Autodesk Fusion 360 part; units mm, degrees
note: some values were not read from the file. Set by a fixed rule: which sketch regions a step uses.
(part 2 of 59)
  spline S4 degree 5 poles (13.0527, -15.6181) (13.0525, -15.6154) (13.0521, -15.61) (13.0515, -15.6019) (13.0506, -15.5911) (13.0495, -15.5777) (13.0484, -15.5644) (13.0473, -15.551) (13.0462, -15.5377) (13.0451, -15.5244) (13.0439, -15.5112) (13.0427, -15.4979) (13.0415, -15.4848) (13.0404, -15.4716) (13.0391, -15.4585) (13.0379, -15.4454) (13.0367, -15.4323) (13.0354, -15.4193) (13.0342, -15.4063) (13.0329, -15.3934) (13.0316, -15.3805) (13.0303, -15.3676) (13.029, -15.3547) (13.0276, -15.3419) (13.0263, -15.3291) (13.0249, -15.3164) (13.0236, -15.3037) (13.0222, -15.291) (13.0208, -15.2784) (13.0194, -15.2658) (13.018, -15.2532) (13.0165, -15.2406) (13.0151, -15.2281) (13.0136, -15.2157) (13.0122, -15.2032) (13.0107, -15.1908) (13.0092, -15.1785) (13.0077, -15.1661) (13.0062, -15.1539) (13.0047, -15.1416) (13.0031, -15.1294) (13.0016, -15.1172) (13, -15.105) (12.9984, -15.0929) (12.9968, -15.0809) (12.9952, -15.0688) (12.9936, -15.0568) (12.992, -15.0449) (12.9904, -15.0329) (12.9887, -15.021) (12.9871, -15.0092) (12.9854, -14.9974) (12.9838, -14.9856) (12.9821, -14.9738) (12.9804, -14.9621) (12.9787, -14.9505) (12.977, -14.9388) (12.9752, -14.9273) (12.9735, -14.9157) (12.9718, -14.9042) (12.97, -14.8927) (12.9682, -14.8813) (12.9665, -14.8699) (12.9647, -14.8585) (12.9629, -14.8472) (12.9611, -14.8359) (12.9593, -14.8247) (12.9574, -14.8135) (12.9556, -14.8023) (12.9538, -14.7912) (12.9519, -14.7801) (12.9501, -14.7691) (12.9482, -14.7581) (12.9463, -14.7471) (12.9445, -14.7362) (12.9426, -14.7253) (12.9407, -14.7145) (12.9388, -14.7037) (12.9368, -14.6929) (12.9349, -14.6822) (12.933, -14.6715) (12.9311, -14.6609) (12.9291, -14.6503) (12.9272, -14.6397) (12.9252, -14.6292) (12.9232, -14.6188) (12.9213, -14.6083) (12.9193, -14.5979) (12.9173, -14.5876) (12.9153, -14.5773) (12.9133, -14.5671) (12.9113, -14.5568) (12.9093, -14.5467) (12.9072, -14.5365) (12.9052, -14.5265) (12.9032, -14.5164) (12.9011, -14.5064) (12.8991, -14.4965) (12.8971, -14.4866) (12.895, -14.4767) (12.8929, -14.4669) (12.8909, -14.4571) (12.8888, -14.4474) (12.8867, -14.4377) (12.8847, -14.4281) (12.8826, -14.4185) (12.8805, -14.4089) (12.8784, -14.3994) (12.8763, -14.39) (12.8742, -14.3806) (12.8721, -14.3712) (12.87, -14.3619) (12.8679, -14.3526) (12.8658, -14.3434) (12.8636, -14.3342) (12.8615, -14.3251) (12.8594, -14.316) (12.8573, -14.3069) (12.8551, -14.298) (12.853, -14.289) (12.8509, -14.2801) (12.8487, -14.2713) (12.8466, -14.2625) (12.8445, -14.2537) (12.8423, -14.2451) (12.8402, -14.2364) (12.838, -14.2278) (12.8359, -14.2193) (12.8337, -14.2108) (12.8316, -14.2023) (12.8294, -14.1939) (12.8273, -14.1856) (12.8251, -14.1773) (12.823, -14.169) (12.8208, -14.1608) (12.8187, -14.1527) (12.8166, -14.1446) (12.8144, -14.1365) (12.8123, -14.1286) (12.8101, -14.1206) (12.808, -14.1127) (12.8058, -14.1049) (12.8037, -14.0971) (12.8016, -14.0894) (12.7994, -14.0817) (12.7973, -14.0741) (12.7952, -14.0665) (12.793, -14.059) (12.7909, -14.0516) (12.7888, -14.0442) (12.7867, -14.0368) (12.7845, -14.0296) (12.7824, -14.0223) (12.7803, -14.0151) (12.7782, -14.008) (12.7761, -14.0009) (12.774, -13.9939) (12.772, -13.987) (12.7699, -13.9801) (12.7678, -13.9733) (12.7657, -13.9665) (12.7637, -13.9598) (12.7616, -13.9531) (12.7596, -13.9465) (12.7575, -13.9399) (12.7555, -13.9335) (12.7534, -13.927) (12.7514, -13.9207) (12.7494, -13.9144) (12.7474, -13.9081) (12.7454, -13.9019) (12.7434, -13.8958) (12.7414, -13.8897) (12.7395, -13.8837) (12.7375, -13.8778) (12.7356, -13.8719) (12.7336, -13.8661) (12.7317, -13.8604) (12.7298, -13.8547) (12.7279, -13.8491) (12.726, -13.8435) (12.7241, -13.838) (12.7222, -13.8326) (12.7204, -13.8273) (12.7185, -13.822) (12.7167, -13.8167) (12.7149, -13.8116) (12.7131, -13.8065) (12.7113, -13.8015) (12.7095, -13.7965) (12.7077, -13.7916) (12.706, -13.7868) (12.7043, -13.782) (12.7026, -13.7774) (12.7009, -13.7728) (12.6992, -13.7682) (12.6975, -13.7638) (12.6959, -13.7594) (12.6943, -13.755) (12.6927, -13.7508) (12.6911, -13.7466) (12.6895, -13.7425) (12.688, -13.7385) (12.6864, -13.7345) (12.6849, -13.7307) (12.6834, -13.7269) (12.682, -13.7231) (12.6806, -13.7195) (12.6791, -13.7159) (12.6778, -13.7124) (12.6764, -13.709) (12.675, -13.7057) (12.6737, -13.7024) (12.6724, -13.6993) (12.6712, -13.6962) (12.6699, -13.6932) (12.6687, -13.6903) (12.6676, -13.6874) (12.6664, -13.6847) (12.6653, -13.682) (12.6642, -13.6794) (12.6631, -13.6769) (12.6621, -13.6745) (12.6611, -13.6722) (12.6602, -13.67) (12.6592, -13.6678) (12.6583, -13.6658) (12.6575, -13.6638) (12.6567, -13.6619) (12.6559, -13.6602) (12.6551, -13.6585) (12.6544, -13.6569) (12.6538, -13.6554) (12.6531, -13.654) (12.6526, -13.6527) (12.652, -13.6515) (12.6515, -13.6504) (12.651, -13.6495) (12.6506, -13.6486) (12.6503, -13.6478) (12.65, -13.6471) (12.6497, -13.6467) (12.6496, -13.6464) (12.6495, -13.6462) (12.6495, -13.6461) knots -1 -1 -1 -1 -1 -1 -0.99583333 -0.99166667 -0.9875 -0.98333333 -0.97916667 -0.975 -0.97083333 -0.96666667 -0.9625 -0.95833333 -0.95416667 -0.95 -0.94583333 -0.94166667 -0.9375 -0.93333333 -0.92916667 -0.925 -0.92083333 -0.91666667 -0.9125 -0.90833333 -0.90416667 -0.9 -0.89583333 -0.89166667 -0.8875 -0.88333333 -0.87916667 -0.875 -0.87083333 -0.86666667 -0.8625 -0.85833333 -0.85416667 -0.85 -0.84583333 -0.84166667 -0.8375 -0.83333333 -0.82916667 -0.825 -0.82083333 -0.81666667 -0.8125 -0.80833333 -0.80416667 -0.8 -0.79583333 -0.79166667 -0.7875 -0.78333333 -0.77916667 -0.775 -0.77083333 -0.76666667 -0.7625 -0.75833333 -0.75416667 -0.75 -0.74583333 -0.74166667 -0.7375 -0.73333333 -0.72916667 -0.725 -0.72083333 -0.71666667 -0.7125 -0.70833333 -0.70416667 -0.7 -0.69583333 -0.69166667 -0.6875 -0.68333333 -0.67916667 -0.675 -0.67083333 -0.66666667 -0.6625 -0.65833333 -0.65416667 -0.65 -0.64583333 -0.64166667 -0.6375 -0.63333333 -0.62916667 -0.625 -0.62083333 -0.61666667 -0.6125 -0.60833333 -0.60416667 -0.6 -0.59583333 -0.59166667 -0.5875 -0.58333333 -0.57916667 -0.575 -0.57083333 -0.56666667 -0.5625 -0.55833333 -0.55416667 -0.55 -0.54583333 -0.54166667 -0.5375 -0.53333333 -0.52916667 -0.525 -0.52083333 -0.51666667 -0.5125 -0.50833333 -0.50416667 -0.5 -0.49583333 -0.49166667 -0.4875 -0.48333333 -0.47916667 -0.475 -0.47083333 -0.46666667 -0.4625 -0.45833333 -0.45416667 -0.45 -0.44583333 -0.44166667 -0.4375 -0.43333333 -0.42916667 -0.425 -0.42083333 -0.41666667 -0.4125 -0.40833333 -0.40416667 -0.4 -0.39583333 -0.39166667 -0.3875 -0.38333333 -0.37916667 -0.375 -0.37083333 -0.36666667 -0.3625 -0.35833333 -0.35416667 -0.35 -0.34583333 -0.34166667 -0.3375 -0.33333333 -0.32916667 -0.325 -0.32083333 -0.31666667 -0.3125 -0.30833333 -0.30416667 -0.3 -0.29583333 -0.29166667 -0.2875 -0.28333333 -0.27916667 -0.275 -0.27083333 -0.26666667 -0.2625 -0.25833333 -0.25416667 -0.25 -0.24583333 -0.24166667 -0.2375 -0.23333333 -0.22916667 -0.225 -0.22083333 -0.21666667 -0.2125 -0.20833333 -0.20416667 -0.2 -0.19583333 -0.19166667 -0.1875 -0.18333333 -0.17916667 -0.175 -0.17083333 -0.16666667 -0.1625 -0.15833333 -0.15416667 -0.15 -0.14583333 -0.14166667 -0.1375 -0.13333333 -0.12916667 -0.125 -0.12083333 -0.11666667 -0.1125 -0.10833333 -0.10416667 -0.1 -0.09583333 -0.09166667 -0.0875 -0.08333333 -0.07916667 -0.075 -0.07083333 -0.06666667 -0.0625 -0.05833333 -0.05416667 -0.05 -0.04583333 -0.04166667 -0.0375 -0.03333333 -0.02916667 -0.025 -0.02083333 -0.01666667 -0.0125 -0.00833333 -0.00416667 0 0 0 0 0 0
  arc A17 (-21.9649, 31.0501) -> (-22.7115, 30.1281) centre (0, 12.5) ccw
  line L24 (23.7836, 28.6526) -> (24.0271, 28.818)
  line L25 (26.1453, 25.1491) -> (25.8803, 25.0209)
  spline S5 degree 5 poles (-9.1146, -17.1298) (-9.1129, -17.1276) (-9.1096, -17.1234) (-9.1047, -17.1169) (-9.0981, -17.1084) (-9.09, -17.0977) (-9.0818, -17.087) (-9.0737, -17.0763) (-9.0657, -17.0657) (-9.0576, -17.055) (-9.0496, -17.0444) (-9.0416, -17.0338) (-9.0337, -17.0232) (-9.0258, -17.0127) (-9.0179, -17.0021) (-9.0101, -16.9915) (-9.0022, -16.981) (-8.9945, -16.9705) (-8.9867, -16.96) (-8.979, -16.9495) (-8.9713, -16.9391) (-8.9637, -16.9286) (-8.956, -16.9182) (-8.9485, -16.9078) (-8.9409, -16.8974) (-8.9334, -16.887) (-8.9259, -16.8766) (-8.9184, -16.8663) (-8.911, -16.856) (-8.9036, -16.8457) (-8.8963, -16.8354) (-8.8889, -16.8251) (-8.8816, -16.8148) (-8.8744, -16.8046) (-8.8671, -16.7944) (-8.86, -16.7842) (-8.8528, -16.774) (-8.8457, -16.7638) (-8.8386, -16.7537) (-8.8315, -16.7435) (-8.8245, -16.7334) (-8.8175, -16.7233) (-8.8105, -16.7132) (-8.8036, -16.7032) (-8.7967, -16.6932) (-8.7898, -16.6831) (-8.783, -16.6731) (-8.7762, -16.6632) (-8.7694, -16.6532) (-8.7626, -16.6433) (-8.7559, -16.6334) (-8.7493, -16.6235) (-8.7426, -16.6136) (-8.736, -16.6037) (-8.7295, -16.5939) (-8.7229, -16.5841) (-8.7164, -16.5743) (-8.7099, -16.5646) (-8.7035, -16.5548) (-8.6971, -16.5451) (-8.6907, -16.5354) (-8.6844, -16.5257) (-8.6781, -16.516) (-8.6718, -16.5064) (-8.6656, -16.4968) (-8.6593, -16.4872) (-8.6532, -16.4776) (-8.647, -16.4681) (-8.6409, -16.4586) (-8.6348, -16.4491) (-8.6288, -16.4396) (-8.6228, -16.4302) (-8.6168, -16.4207) (-8.6109, -16.4113) (-8.605, -16.402) (-8.5991, -16.3926) (-8.5932, -16.3833) (-8.5874, -16.374) (-8.5817, -16.3647) (-8.5759, -16.3555) (-8.5702, -16.3462) (-8.5645, -16.337) (-8.5589, -16.3279) (-8.5533, -16.3187) (-8.5477, -16.3096) (-8.5422, -16.3005) (-8.5367, -16.2914) (-8.5312, -16.2824) (-8.5257, -16.2734) (-8.5203, -16.2644) (-8.515, -16.2554) (-8.5096, -16.2465) (-8.5043, -16.2376) (-8.499, -16.2287) (-8.4938, -16.2199) (-8.4886, -16.211) (-8.4834, -16.2022) (-8.4783, -16.1935) (-8.4732, -16.1847) (-8.4681, -16.176) (-8.463, -16.1674) (-8.458, -16.1587) (-8.4531, -16.1501) (-8.4481, -16.1415) (-8.4432, -16.133) (-8.4384, -16.1244) (-8.4335, -16.116) (-8.4287, -16.1075) (-8.4239, -16.0991) (-8.4192, -16.0907) (-8.4145, -16.0823) (-8.4098, -16.074) (-8.4052, -16.0657) (-8.4006, -16.0574) (-8.396, -16.0491) (-8.3915, -16.0409) (-8.387, -16.0328) (-8.3825, -16.0246) (-8.3781, -16.0165) (-8.3737, -16.0085) (-8.3693, -16.0004) (-8.365, -15.9924) (-8.3607, -15.9845) (-8.3565, -15.9765) (-8.3522, -15.9686) (-8.348, -15.9608) (-8.3439, -15.9529) (-8.3398, -15.9452) (-8.3357, -15.9374) (-8.3316, -15.9297) (-8.3276, -15.922) (-8.3236, -15.9144) (-8.3196, -15.9068) (-8.3157, -15.8992) (-8.3118, -15.8917) (-8.308, -15.8842) (-8.3042, -15.8767) (-8.3004, -15.8693) (-8.2966, -15.8619) (-8.2929, -15.8546) (-8.2892, -15.8473) (-8.2856, -15.8401) (-8.282, -15.8329) (-8.2784, -15.8257) (-8.2748, -15.8186) (-8.2713, -15.8115) (-8.2678, -15.8044) (-8.2644, -15.7974) (-8.261, -15.7905) (-8.2576, -15.7835) (-8.2543, -15.7767) (-8.251, -15.7698) (-8.2477, -15.763) (-8.2445, -15.7563) (-8.2412, -15.7496) (-8.2381, -15.7429) (-8.2349, -15.7363) (-8.2318, -15.7298) (-8.2288, -15.7233) (-8.2257, -15.7168) (-8.2227, -15.7104) (-8.2198, -15.704) (-8.2169, -15.6977) (-8.214, -15.6914) (-8.2111, -15.6851) (-8.2083, -15.679) (-8.2055, -15.6728) (-8.2027, -15.6667) (-8.2, -15.6607) (-8.1973, -15.6547) (-8.1947, -15.6488) (-8.192, -15.6429) (-8.1895, -15.6371) (-8.1869, -15.6313) (-8.1844, -15.6256) (-8.1819, -15.6199) (-8.1795, -15.6143) (-8.177, -15.6087) (-8.1747, -15.6032) (-8.1723, -15.5978) (-8.17, -15.5924) (-8.1677, -15.587) (-8.1655, -15.5818) (-8.1633, -15.5765) (-8.1611, -15.5714) (-8.159, -15.5663) (-8.1569, -15.5612) (-8.1548, -15.5562) (-8.1528, -15.5513) (-8.1508, -15.5464) (-8.1488, -15.5416) (-8.1469, -15.5369) (-8.145, -15.5322) (-8.1432, -15.5276) (-8.1413, -15.523) (-8.1395, -15.5185) (-8.1378, -15.5141) (-8.1361, -15.5097) (-8.1344, -15.5054) (-8.1327, -15.5012) (-8.1311, -15.497) (-8.1295, -15.4929) (-8.128, -15.4889) (-8.1265, -15.4849) (-8.125, -15.4811) (-8.1236, -15.4772) (-8.1222, -15.4735) (-8.1208, -15.4698) (-8.1194, -15.4662) (-8.1181, -15.4627) (-8.1169, -15.4593) (-8.1156, -15.4559) (-8.1144, -15.4526) (-8.1133, -15.4494) (-8.1121, -15.4462) (-8.1111, -15.4432) (-8.11, -15.4402) (-8.109, -15.4373) (-8.108, -15.4345) (-8.107, -15.4318) (-8.1061, -15.4291) (-8.1052, -15.4265) (-8.1044, -15.4241) (-8.1036, -15.4217) (-8.1028, -15.4194) (-8.102, -15.4172) (-8.1013, -15.415) (-8.1007, -15.413) (-8.1, -15.4111) (-8.0994, -15.4092) (-8.0988, -15.4075) (-8.0983, -15.4058) (-8.0978, -15.4043) (-8.0973, -15.4028) (-8.0969, -15.4015) (-8.0965, -15.4002) (-8.0962, -15.3991) (-8.0958, -15.398) (-8.0956, -15.3971) (-8.0953, -15.3963) (-8.0951, -15.3956) (-8.0949, -15.3951) (-8.0948, -15.3948) (-8.0948, -15.3946) (-8.0948, -15.3945) knots -1 -1 -1 -1 -1 -1 -0.99583333 -0.99166667 -0.9875 -0.98333333 -0.97916667 -0.975 -0.97083333 -0.96666667 -0.9625 -0.95833333 -0.95416667 -0.95 -0.94583333 -0.94166667 -0.9375 -0.93333333 -0.92916667 -0.925 -0.92083333 -0.91666667 -0.9125 -0.90833333 -0.90416667 -0.9 -0.89583333 -0.89166667 -0.8875 -0.88333333 -0.87916667 -0.875 -0.87083333 -0.86666667 -0.8625 -0.85833333 -0.85416667 -0.85 -0.84583333 -0.84166667 -0.8375 -0.83333333 -0.82916667 -0.825 -0.82083333 -0.81666667 -0.8125 -0.80833333 -0.80416667 -0.8 -0.79583333 -0.79166667 -0.7875 -0.78333333 -0.77916667 -0.775 -0.77083333 -0.76666667 -0.7625 -0.75833333 -0.75416667 -0.75 -0.74583333 -0.74166667 -0.7375 -0.73333333 -0.72916667 -0.725 -0.72083333 -0.71666667 -0.7125 -0.70833333 -0.70416667 -0.7 -0.69583333 -0.69166667 -0.6875 -0.68333333 -0.67916667 -0.675 -0.67083333 -0.66666667 -0.6625 -0.65833333 -0.65416667 -0.65 -0.64583333 -0.64166667 -0.6375 -0.63333333 -0.62916667 -0.625 -0.62083333 -0.61666667 -0.6125 -0.60833333 -0.60416667 -0.6 -0.59583333 -0.59166667 -0.5875 -0.58333333 -0.57916667 -0.575 -0.57083333 -0.56666667 -0.5625 -0.55833333 -0.55416667 -0.55 -0.54583333 -0.54166667 -0.5375 -0.53333333 -0.52916667 -0.525 -0.52083333 -0.51666667 -0.5125 -0.50833333 -0.50416667 -0.5 -0.49583333 -0.49166667 -0.4875 -0.48333333 -0.47916667 -0.475 -0.47083333 -0.46666667 -0.4625 -0.45833333 -0.45416667 -0.45 -0.44583333 -0.44166667 -0.4375 -0.43333333 -0.42916667 -0.425 -0.42083333 -0.41666667 -0.4125 -0.40833333 -0.40416667 -0.4 -0.39583333 -0.39166667 -0.3875 -0.38333333 -0.37916667 -0.375 -0.37083333 -0.36666667 -0.3625 -0.35833333 -0.35416667 -0.35 -0.34583333 -0.34166667 -0.3375 -0.33333333 -0.32916667 -0.325 -0.32083333 -0.31666667 -0.3125 -0.30833333 -0.30416667 -0.3 -0.29583333 -0.29166667 -0.2875 -0.28333333 -0.27916667 -0.275 -0.27083333 -0.26666667 -0.2625 -0.25833333 -0.25416667 -0.25 -0.24583333 -0.24166667 -0.2375 -0.23333333 -0.22916667 -0.225 -0.22083333 -0.21666667 -0.2125 -0.20833333 -0.20416667 -0.2 -0.19583333 -0.19166667 -0.1875 -0.18333333 -0.17916667 -0.175 -0.17083333 -0.16666667 -0.1625 -0.15833333 -0.15416667 -0.15 -0.14583333 -0.14166667 -0.1375 -0.13333333 -0.12916667 -0.125 -0.12083333 -0.11666667 -0.1125 -0.10833333 -0.10416667 -0.1 -0.09583333 -0.09166667 -0.0875 -0.08333333 -0.07916667 -0.075 -0.07083333 -0.06666667 -0.0625 -0.05833333 -0.05416667 -0.05 -0.04583333 -0.04166667 -0.0375 -0.03333333 -0.02916667 -0.025 -0.02083333 -0.01666667 -0.0125 -0.00833333 -0.00416667 0 0 0 0 0 0
  arc A18 (27.0473, 22.2471) -> (26.6221, 23.3547) centre (0, 12.5) ccw
  spline S6 degree 5 poles (13.7175, -13.1019) (13.7175, -13.102) (13.7176, -13.1022) (13.7178, -13.1025) (13.718, -13.1029) (13.7184, -13.1036) (13.7188, -13.1043) (13.7193, -13.1052) (13.7198, -13.1061) (13.7204, -13.1072) (13.721, -13.1083) (13.7217, -13.1096) (13.7225, -13.1109) (13.7233, -13.1123) (13.7242, -13.1138) (13.7251, -13.1154) (13.7261, -13.1171) (13.7271, -13.1188) (13.7282, -13.1207) (13.7293, -13.1226) (13.7305, -13.1246) (13.7317, -13.1267) (13.733, -13.1289) (13.7344, -13.1311) (13.7358, -13.1334) (13.7372, -13.1358) (13.7387, -13.1383) (13.7403, -13.1409) (13.7419, -13.1435) (13.7435, -13.1462) (13.7452, -13.1489) (13.747, -13.1518) (13.7488, -13.1547) (13.7506, -13.1577) (13.7526, -13.1607) (13.7545, -13.1638) (13.7565, -13.167) (13.7586, -13.1702) (13.7607, -13.1735) (13.7628, -13.1769) (13.765, -13.1803) (13.7673, -13.1838) (13.7696, -13.1874) (13.7719, -13.191) (13.7743, -13.1947) (13.7768, -13.1984) (13.7793, -13.2022) (13.7818, -13.206) (13.7844, -13.21) (13.787, -13.2139) (13.7897, -13.218) (13.7925, -13.222) (13.7952, -13.2262) (13.7981, -13.2304) (13.8009, -13.2346) (13.8039, -13.2389) (13.8068, -13.2432) (13.8098, -13.2476) (13.8129, -13.2521) (13.816, -13.2566) (13.8192, -13.2612) (13.8224, -13.2658) (13.8256, -13.2704) (13.8289, -13.2751) (13.8322, -13.2799) (13.8356, -13.2847) (13.839, -13.2895) (13.8425, -13.2944) (13.846, -13.2993) (13.8496, -13.3043) (13.8532, -13.3093) (13.8568, -13.3144) (13.8605, -13.3195) (13.8643, -13.3247) (13.8681, -13.3299) (13.8719, -13.3352) (13.8758, -13.3405) (13.8797, -13.3458) (13.8836, -13.3512) (13.8876, -13.3566) (13.8917, -13.3621) (13.8958, -13.3676) (13.8999, -13.3731) (13.9041, -13.3787) (13.9083, -13.3843) (13.9126, -13.39) (13.9169, -13.3957) (13.9213, -13.4014) (13.9257, -13.4072) (13.9301, -13.413) (13.9346, -13.4188) (13.9391, -13.4247) (13.9437, -13.4306) (13.9483, -13.4366) (13.9529, -13.4426) (13.9576, -13.4486) (13.9624, -13.4547) (13.9672, -13.4608) (13.972, -13.4669) (13.9769, -13.4731) (13.9818, -13.4793) (13.9867, -13.4855) (13.9917, -13.4918) (13.9967, -13.4981) (14.0018, -13.5044) (14.0069, -13.5108) (14.0121, -13.5172) (14.0173, -13.5236) (14.0225, -13.5301) (14.0278, -13.5366) (14.0332, -13.5431) (14.0385, -13.5497) (14.0439, -13.5563) (14.0494, -13.5629) (14.0549, -13.5695) (14.0604, -13.5762) (14.066, -13.5829) (14.0716, -13.5896) (14.0772, -13.5964) (14.0829, -13.6032) (14.0887, -13.61) (14.0945, -13.6168) (14.1003, -13.6237) (14.1061, -13.6306) (14.112, -13.6375) (14.118, -13.6445) (14.1239, -13.6515) (14.13, -13.6585) (14.136, -13.6655) (14.1421, -13.6726) (14.1483, -13.6796) (14.1544, -13.6868) (14.1607, -13.6939) (14.1669, -13.701) (14.1732, -13.7082) (14.1796, -13.7154) (14.1859, -13.7227) (14.1924, -13.7299) (14.1988, -13.7372) (14.2053, -13.7445) (14.2119, -13.7518) (14.2184, -13.7592) (14.225, -13.7665) (14.2317, -13.7739) (14.2384, -13.7813) (14.2451, -13.7888) (14.2519, -13.7962) (14.2587, -13.8037) (14.2656, -13.8112) (14.2724, -13.8188) (14.2794, -13.8263) (14.2863, -13.8339) (14.2933, -13.8414) (14.3004, -13.8491) (14.3075, -13.8567) (14.3146, -13.8643) (14.3217, -13.872) (14.3289, -13.8797) (14.3362, -13.8874) (14.3435, -13.8951) (14.3508, -13.9029) (14.3581, -13.9106) (14.3655, -13.9184) (14.3729, -13.9262) (14.3804, -13.934) (14.3879, -13.9419) (14.3954, -13.9497) (14.403, -13.9576) (14.4106, -13.9655) (14.4183, -13.9734) (14.426, -13.9813) (14.4337, -13.9893) (14.4415, -13.9972) (14.4493, -14.0052) (14.4571, -14.0132) (14.465, -14.0212) (14.4729, -14.0292) (14.4809, -14.0373) (14.4889, -14.0453) (14.4969, -14.0534) (14.505, -14.0615) (14.5131, -14.0696) (14.5212, -14.0777) (14.5294, -14.0858) (14.5376, -14.094) (14.5459, -14.1022) (14.5541, -14.1103) (14.5625, -14.1185) (14.5708, -14.1267) (14.5792, -14.135) (14.5877, -14.1432) (14.5961, -14.1514) (14.6046, -14.1597) (14.6132, -14.168) (14.6218, -14.1763) (14.6304, -14.1846) (14.639, -14.1929) (14.6477, -14.2012) (14.6565, -14.2096) (14.6652, -14.2179) (14.674, -14.2263) (14.6829, -14.2347) (14.6917, -14.2431) (14.7006, -14.2515) (14.7096, -14.2599) (14.7186, -14.2683) (14.7276, -14.2767) (14.7366, -14.2852) (14.7457, -14.2937) (14.7549, -14.3021) (14.764, -14.3106) (14.7732, -14.3191) (14.7824, -14.3276) (14.7917, -14.3361) (14.801, -14.3447) (14.8104, -14.3532) (14.8197, -14.3618) (14.8291, -14.3703) (14.8386, -14.3789) (14.8481, -14.3875) (14.8576, -14.3961) (14.8671, -14.4047) (14.8767, -14.4133) (14.8863, -14.4219) (14.896, -14.4305) (14.9057, -14.4392) (14.9154, -14.4478) (14.9252, -14.4565) (14.935, -14.4651) (14.9448, -14.4738) (14.9547, -14.4825) (14.9646, -14.4912) (14.9745, -14.4999) (14.9845, -14.5086) (14.9945, -14.5173) (15.0045, -14.526) (15.0146, -14.5347) (15.0247, -14.5435) (15.0349, -14.5522) (15.045, -14.561) (15.0553, -14.5697) (15.0635, -14.5767) (15.0696, -14.582) (15.0737, -14.5855) (15.0758, -14.5873) knots 0 0 0 0 0 0 0.00416667 0.00833333 0.0125 0.01666667 0.02083333 0.025 0.02916667 0.03333333 0.0375 0.04166667 0.04583333 0.05 0.05416667 0.05833333 0.0625 0.06666667 0.07083333 0.075 0.07916667 0.08333333 0.0875 0.09166667 0.09583333 0.1 0.10416667 0.10833333 0.1125 0.11666667 0.12083333 0.125 0.12916667 0.13333333 0.1375 0.14166667 0.14583333 0.15 0.15416667 0.15833333 0.1625 0.16666667 0.17083333 0.175 0.17916667 0.18333333 0.1875 0.19166667 0.19583333 0.2 0.20416667 0.20833333 0.2125 0.21666667 0.22083333 0.225 0.22916667 0.23333333 0.2375 0.24166667 0.24583333 0.25 0.25416667 0.25833333 0.2625 0.26666667 0.27083333 0.275 0.27916667 0.28333333 0.2875 0.29166667 0.29583333 0.3 0.30416667 0.30833333 0.3125 0.31666667 0.32083333 0.325 0.32916667 0.33333333 0.3375 0.34166667 0.34583333 0.35 0.35416667 0.35833333 0.3625 0.36666667 0.37083333 0.375 0.37916667 0.38333333 0.3875 0.39166667 0.39583333 0.4 0.40416667 0.40833333 0.4125 0.41666667 0.42083333 0.425 0.42916667 0.43333333 0.4375 0.44166667 0.44583333 0.45 0.45416667 0.45833333 0.4625 0.46666667 0.47083333 0.475 0.47916667 0.48333333 0.4875 0.49166667 0.49583333 0.5 0.50416667 0.50833333 0.5125 0.51666667 0.52083333 0.525 0.52916667 0.53333333 0.5375 0.54166667 0.54583333 0.55 0.55416667 0.55833333 0.5625 0.56666667 0.57083333 0.575 0.57916667 0.58333333 0.5875 0.59166667 0.59583333 0.6 0.60416667 0.60833333 0.6125 0.61666667 0.62083333 0.625 0.62916667 0.63333333 0.6375 0.64166667 0.64583333 0.65 0.65416667 0.65833333 0.6625 0.66666667 0.67083333 0.675 0.67916667 0.68333333 0.6875 0.69166667 0.69583333 0.7 0.70416667 0.70833333 0.7125 0.71666667 0.72083333 0.725 0.72916667 0.73333333 0.7375 0.74166667 0.74583333 0.75 0.75416667 0.75833333 0.7625 0.76666667 0.77083333 0.775 0.77916667 0.78333333 0.7875 0.79166667 0.79583333 0.8 0.80416667 0.80833333 0.8125 0.81666667 0.82083333 0.825 0.82916667 0.83333333 0.8375 0.84166667 0.84583333 0.85 0.85416667 0.85833333 0.8625 0.86666667 0.87083333 0.875 0.87916667 0.88333333 0.8875 0.89166667 0.89583333 0.9 0.90416667 0.90833333 0.9125 0.91666667 0.92083333 0.925 0.92916667 0.93333333 0.9375 0.94166667 0.94583333 0.95 0.95416667 0.95833333 0.9625 0.96666667 0.97083333 0.975 0.97916667 0.98333333 0.9875 0.99166667 0.99583333 1 1 1 1 1 1
  line L26 (25.6012, 26.2171) -> (25.6019, 26.2175)
  arc A19 (28.5147, 24.6618) -> (28.1181, 25.5527) centre (0, 12.5) ccw
  line L27 (28.5878, 7.3654) -> (28.587, 7.3655)
  arc A20 (28.2972, 7.4176) -> (28.4828, 8.5894) centre (0, 12.5) ccw
  spline S7 degree 5 poles (28.2047, 5.563) (28.2048, 5.563) (28.205, 5.563) (28.2053, 5.5629) (28.2058, 5.5628) (28.2065, 5.5626) (28.2074, 5.5624) (28.2083, 5.5622) (28.2094, 5.5619) (28.2106, 5.5617) (28.2118, 5.5614) (28.2132, 5.5611) (28.2147, 5.5608) (28.2163, 5.5604) (28.218, 5.5601) (28.2198, 5.5597) (28.2217, 5.5593) (28.2237, 5.5589) (28.2258, 5.5584) (28.228, 5.558) (28.2303, 5.5575) (28.2327, 5.5571) (28.2351, 5.5566) (28.2377, 5.5561) (28.2404, 5.5555) (28.2431, 5.555) (28.246, 5.5545) (28.2489, 5.5539) (28.2519, 5.5534) (28.255, 5.5528) (28.2582, 5.5522) (28.2615, 5.5516) (28.2649, 5.551) (28.2683, 5.5504) (28.2719, 5.5498) (28.2755, 5.5492) (28.2792, 5.5485) (28.283, 5.5479) (28.2868, 5.5472) (28.2908, 5.5466) (28.2948, 5.5459) (28.2989, 5.5453) (28.3031, 5.5446) (28.3074, 5.5439) (28.3117, 5.5432) (28.3161, 5.5426) (28.3206, 5.5419) (28.3252, 5.5412) (28.3298, 5.5405) (28.3345, 5.5398) (28.3393, 5.5391) (28.3442, 5.5384) (28.3491, 5.5377) (28.3541, 5.537) (28.3592, 5.5363) (28.3643, 5.5356) (28.3695, 5.5349) (28.3748, 5.5342) (28.3802, 5.5335) (28.3856, 5.5328) (28.3911, 5.5321) (28.3966, 5.5314) (28.4023, 5.5307) (28.408, 5.53) (28.4137, 5.5293) (28.4196, 5.5286) (28.4255, 5.5279) (28.4314, 5.5272) (28.4374, 5.5265) (28.4435, 5.5258) (28.4497, 5.5251) (28.4559, 5.5244) (28.4622, 5.5237) (28.4685, 5.5231) (28.4749, 5.5224) (28.4814, 5.5217) (28.4879, 5.5211) (28.4945, 5.5204) (28.5011, 5.5197) (28.5078, 5.5191) (28.5146, 5.5184) (28.5214, 5.5178) (28.5283, 5.5172) (28.5353, 5.5165) (28.5423, 5.5159) (28.5493, 5.5153) (28.5564, 5.5147) (28.5636, 5.5141) (28.5709, 5.5135) (28.5781, 5.5129) (28.5855, 5.5123) (28.5929, 5.5118) (28.6004, 5.5112) (28.6079, 5.5106) (28.6154, 5.5101) (28.6231, 5.5095) (28.6307, 5.509) (28.6385, 5.5085) (28.6463, 5.5079) (28.6541, 5.5074) (28.662, 5.5069) (28.67, 5.5064) (28.678, 5.506) (28.686, 5.5055) (28.6941, 5.505) (28.7023, 5.5046) (28.7105, 5.5041) (28.7187, 5.5037) (28.727, 5.5032) (28.7354, 5.5028) (28.7438, 5.5024) (28.7523, 5.502) (28.7608, 5.5016) (28.7694, 5.5013) (28.778, 5.5009) (28.7866, 5.5005) (28.7953, 5.5002) (28.8041, 5.4999) (28.8129, 5.4995) (28.8218, 5.4992) (28.8307, 5.4989) (28.8396, 5.4986) (28.8486, 5.4984) (28.8577, 5.4981) (28.8668, 5.4979) (28.8759, 5.4976) (28.8851, 5.4974) (28.8943, 5.4972) (28.9036, 5.497) (28.9129, 5.4968) (28.9223, 5.4966) (28.9317, 5.4964) (28.9412, 5.4963) (28.9507, 5.4962) (28.9602, 5.496) (28.9698, 5.4959) (28.9795, 5.4958) (28.9892, 5.4957) (28.9989, 5.4957) (29.0087, 5.4956) (29.0185, 5.4956) (29.0284, 5.4955) (29.0383, 5.4955) (29.0482, 5.4955) (29.0582, 5.4955) (29.0682, 5.4956) (29.0783, 5.4956) (29.0884, 5.4957) (29.0986, 5.4957) (29.1088, 5.4958) (29.119, 5.4959) (29.1293, 5.496) (29.1396, 5.4962) (29.15, 5.4963) (29.1604, 5.4965) (29.1708, 5.4966) (29.1813, 5.4968) (29.1919, 5.497) (29.2024, 5.4972) (29.213, 5.4975) (29.2237, 5.4977) (29.2344, 5.498) (29.2451, 5.4983) (29.2559, 5.4986) (29.2667, 5.4989) (29.2775, 5.4992) (29.2884, 5.4996) (29.2993, 5.4999) (29.3103, 5.5003) (29.3213, 5.5007) (29.3323, 5.5011) (29.3434, 5.5016) (29.3545, 5.502) (29.3657, 5.5025) (29.3768, 5.503) (29.3881, 5.5035) (29.3993, 5.504) (29.4106, 5.5045) (29.422, 5.505) (29.4333, 5.5056) (29.4447, 5.5062) (29.4562, 5.5068) (29.4677, 5.5074) (29.4792, 5.508) (29.4907, 5.5087) (29.5023, 5.5094) (29.514, 5.51) (29.5256, 5.5108) (29.5373, 5.5115) (29.549, 5.5122) (29.5608, 5.513) (29.5726, 5.5137) (29.5844, 5.5145) (29.5963, 5.5154) (29.6082, 5.5162) (29.6201, 5.517) (29.6321, 5.5179) (29.6441, 5.5188) (29.6562, 5.5197) (29.6682, 5.5206) (29.6803, 5.5216) (29.6925, 5.5225) (29.7047, 5.5235) (29.7169, 5.5245) (29.7291, 5.5255) (29.7414, 5.5265) (29.7537, 5.5276) (29.766, 5.5287) (29.7784, 5.5298) (29.7908, 5.5309) (29.8032, 5.532) (29.8157, 5.5331) (29.8282, 5.5343) (29.8407, 5.5355) (29.8533, 5.5367) (29.8659, 5.5379) (29.8785, 5.5392) (29.8912, 5.5404) (29.9039, 5.5417) (29.9166, 5.543) (29.9293, 5.5444) (29.9421, 5.5457) (29.9549, 5.5471) (29.9678, 5.5484) (29.9806, 5.5499) (29.9935, 5.5513) (30.0065, 5.5527) (30.0194, 5.5542) (30.0324, 5.5557) (30.0455, 5.5572) (30.0585, 5.5587) (30.0716, 5.5602) (30.0847, 5.5618) (30.0979, 5.5634) (30.111, 5.565) (30.1242, 5.5666) (30.1375, 5.5683) (30.1507, 5.5699) (30.164, 5.5716) (30.1773, 5.5733) (30.1907, 5.575) (30.2014, 5.5764) (30.2094, 5.5775) (30.2148, 5.5782) (30.2174, 5.5786) knots 0 0 0 0 0 0 0.00416667 0.00833333 0.0125 0.01666667 0.02083333 0.025 0.02916667 0.03333333 0.0375 0.04166667 0.04583333 0.05 0.05416667 0.05833333 0.0625 0.06666667 0.07083333 0.075 0.07916667 0.08333333 0.0875 0.09166667 0.09583333 0.1 0.10416667 0.10833333 0.1125 0.11666667 0.12083333 0.125 0.12916667 0.13333333 0.1375 0.14166667 0.14583333 0.15 0.15416667 0.15833333 0.1625 0.16666667 0.17083333 0.175 0.17916667 0.18333333 0.1875 0.19166667 0.19583333 0.2 0.20416667 0.20833333 0.2125 0.21666667 0.22083333 0.225 0.22916667 0.23333333 0.2375 0.24166667 0.24583333 0.25 0.25416667 0.25833333 0.2625 0.26666667 0.27083333 0.275 0.27916667 0.28333333 0.2875 0.29166667 0.29583333 0.3 0.30416667 0.30833333 0.3125 0.31666667 0.32083333 0.325 0.32916667 0.33333333 0.3375 0.34166667 0.34583333 0.35 0.35416667 0.35833333 0.3625 0.36666667 0.37083333 0.375 0.37916667 0.38333333 0.3875 0.39166667 0.39583333 0.4 0.40416667 0.40833333 0.4125 0.41666667 0.42083333 0.425 0.42916667 0.43333333 0.4375 0.44166667 0.44583333 0.45 0.45416667 0.45833333 0.4625 0.46666667 0.47083333 0.475 0.47916667 0.48333333 0.4875 0.49166667 0.49583333 0.5 0.50416667 0.50833333 0.5125 0.51666667 0.52083333 0.525 0.52916667 0.53333333 0.5375 0.54166667 0.54583333 0.55 0.55416667 0.55833333 0.5625 0.56666667 0.57083333 0.575 0.57916667 0.58333333 0.5875 0.59166667 0.59583333 0.6 0.60416667 0.60833333 0.6125 0.61666667 0.62083333 0.625 0.62916667 0.63333333 0.6375 0.64166667 0.64583333 0.65 0.65416667 0.65833333 0.6625 0.66666667 0.67083333 0.675 0.67916667 0.68333333 0.6875 0.69166667 0.69583333 0.7 0.70416667 0.70833333 0.7125 0.71666667 0.72083333 0.725 0.72916667 0.73333333 0.7375 0.74166667 0.74583333 0.75 0.75416667 0.75833333 0.7625 0.76666667 0.77083333 0.775 0.77916667 0.78333333 0.7875 0.79166667 0.79583333 0.8 0.80416667 0.80833333 0.8125 0.81666667 0.82083333 0.825 0.82916667 0.83333333 0.8375 0.84166667 0.84583333 0.85 0.85416667 0.85833333 0.8625 0.86666667 0.87083333 0.875 0.87916667 0.88333333 0.8875 0.89166667 0.89583333 0.9 0.90416667 0.90833333 0.9125 0.91666667 0.92083333 0.925 0.92916667 0.93333333 0.9375 0.94166667 0.94583333 0.95 0.95416667 0.95833333 0.9625 0.96666667 0.97083333 0.975 0.97916667 0.98333333 0.9875 0.99166667 0.99583333 1 1 1 1 1 1
  line L28 (5.1345, 41.087) -> (5.0824, 40.7972)
  line L29 (-0.9213, -16.5298) -> (-0.9213, -16.5307)
  line L30 (9.8472, -14.8251) -> (9.8469, -14.8243)
  arc A21 (30.2174, 5.5786) -> (30.4202, 6.5325) centre (0, 12.5) ccw
  line L31 (28.6734, 14.5967) -> (28.9671, 14.6182)
  line L32 (6.9368, 40.7039) -> (6.937, 40.7047)
  line L33 (6.8665, 40.418) -> (6.9368, 40.7039)
  line L34 (-2.1183, -16.4679) -> (-2.1182, -16.4671)
  line L35 (28.9671, 14.6182) -> (28.9679, 14.6183)
  arc A22 (5.9675, -17.9202) -> (6.9214, -17.7174) centre (0, 12.5) ccw
  line L36 (8.0125, -15.1109) -> (8.0945, -15.3937)
  line L37 (8.0945, -15.3937) -> (8.0948, -15.3945)
  line L38 (-2.1182, -16.4671) -> (-2.0967, -16.1734)
  spline S8 degree 5 poles (29.6298, 3.3854) (29.6276, 3.3871) (29.6234, 3.3904) (29.6169, 3.3953) (29.6084, 3.4019) (29.5977, 3.41) (29.587, 3.4182) (29.5763, 3.4263) (29.5657, 3.4343) (29.555, 3.4424) (29.5444, 3.4504) (29.5338, 3.4584) (29.5232, 3.4663) (29.5127, 3.4742) (29.5021, 3.4821) (29.4915, 3.4899) (29.481, 3.4978) (29.4705, 3.5055) (29.46, 3.5133) (29.4495, 3.521) (29.4391, 3.5287) (29.4286, 3.5363) (29.4182, 3.544) (29.4078, 3.5515) (29.3974, 3.5591) (29.387, 3.5666) (29.3766, 3.5741) (29.3663, 3.5816) (29.356, 3.589) (29.3457, 3.5964) (29.3354, 3.6037) (29.3251, 3.6111) (29.3148, 3.6184) (29.3046, 3.6256) (29.2944, 3.6329) (29.2842, 3.64) (29.274, 3.6472) (29.2638, 3.6543) (29.2537, 3.6614) (29.2435, 3.6685) (29.2334, 3.6755) (29.2233, 3.6825) (29.2132, 3.6895) (29.2032, 3.6964) (29.1932, 3.7033) (29.1831, 3.7102) (29.1731, 3.717) (29.1632, 3.7238) (29.1532, 3.7306) (29.1433, 3.7374) (29.1334, 3.7441) (29.1235, 3.7507) (29.1136, 3.7574) (29.1037, 3.764) (29.0939, 3.7705) (29.0841, 3.7771) (29.0743, 3.7836) (29.0646, 3.7901) (29.0548, 3.7965) (29.0451, 3.8029) (29.0354, 3.8093) (29.0257, 3.8156) (29.016, 3.8219) (29.0064, 3.8282) (28.9968, 3.8344) (28.9872, 3.8407) (28.9776, 3.8468) (28.9681, 3.853) (28.9586, 3.8591) (28.9491, 3.8652) (28.9396, 3.8712) (28.9302, 3.8772) (28.9207, 3.8832) (28.9113, 3.8891) (28.902, 3.895) (28.8926, 3.9009) (28.8833, 3.9068) (28.874, 3.9126) (28.8647, 3.9183) (28.8555, 3.9241) (28.8462, 3.9298) (28.837, 3.9355) (28.8279, 3.9411) (28.8187, 3.9467) (28.8096, 3.9523) (28.8005, 3.9578) (28.7914, 3.9633) (28.7824, 3.9688) (28.7734, 3.9743) (28.7644, 3.9797) (28.7554, 3.985) (28.7465, 3.9904) (28.7376, 3.9957) (28.7287, 4.001) (28.7199, 4.0062) (28.711, 4.0114) (28.7022, 4.0166) (28.6935, 4.0217) (28.6847, 4.0268) (28.676, 4.0319) (28.6674, 4.037) (28.6587, 4.042) (28.6501, 4.0469) (28.6415, 4.0519) (28.633, 4.0568) (28.6244, 4.0616) (28.616, 4.0665) (28.6075, 4.0713) (28.5991, 4.0761) (28.5907, 4.0808) (28.5823, 4.0855) (28.574, 4.0902) (28.5657, 4.0948) (28.5574, 4.0994) (28.5491, 4.104) (28.5409, 4.1085) (28.5328, 4.113) (28.5246, 4.1175) (28.5165, 4.1219) (28.5085, 4.1263) (28.5004, 4.1307) (28.4924, 4.135) (28.4845, 4.1393) (28.4765, 4.1435) (28.4686, 4.1478) (28.4608, 4.152) (28.4529, 4.1561) (28.4452, 4.1602) (28.4374, 4.1643) (28.4297, 4.1684) (28.422, 4.1724) (28.4144, 4.1764) (28.4068, 4.1804) (28.3992, 4.1843) (28.3917, 4.1882) (28.3842, 4.192) (28.3767, 4.1958) (28.3693, 4.1996) (28.3619, 4.2034) (28.3546, 4.2071) (28.3473, 4.2108) (28.3401, 4.2144) (28.3329, 4.218) (28.3257, 4.2216) (28.3186, 4.2252) (28.3115, 4.2287) (28.3044, 4.2322) (28.2974, 4.2356) (28.2905, 4.239) (28.2835, 4.2424) (28.2767, 4.2457) (28.2698, 4.249) (28.263, 4.2523) (28.2563, 4.2555) (28.2496, 4.2588) (28.2429, 4.2619) (28.2363, 4.2651) (28.2298, 4.2682) (28.2233, 4.2712) (28.2168, 4.2743) (28.2104, 4.2773) (28.204, 4.2802) (28.1977, 4.2831) (28.1914, 4.286) (28.1851, 4.2889) (28.179, 4.2917) (28.1728, 4.2945) (28.1667, 4.2973) (28.1607, 4.3) (28.1547, 4.3027) (28.1488, 4.3053) (28.1429, 4.308) (28.1371, 4.3105) (28.1313, 4.3131) (28.1256, 4.3156) (28.1199, 4.3181) (28.1143, 4.3205) (28.1087, 4.323) (28.1032, 4.3253) (28.0978, 4.3277) (28.0924, 4.33) (28.087, 4.3323) (28.0818, 4.3345) (28.0765, 4.3367) (28.0714, 4.3389) (28.0663, 4.341) (28.0612, 4.3431) (28.0562, 4.3452) (28.0513, 4.3472) (28.0464, 4.3492) (28.0416, 4.3512) (28.0369, 4.3531) (28.0322, 4.355) (28.0276, 4.3568) (28.023, 4.3587) (28.0185, 4.3605) (28.0141, 4.3622) (28.0097, 4.3639) (28.0054, 4.3656) (28.0012, 4.3673) (27.997, 4.3689) (27.9929, 4.3705) (27.9889, 4.372) (27.9849, 4.3735) (27.9811, 4.375) (27.9772, 4.3764) (27.9735, 4.3778) (27.9698, 4.3792) (27.9662, 4.3806) (27.9627, 4.3819) (27.9593, 4.3831) (27.9559, 4.3844) (27.9526, 4.3856) (27.9494, 4.3867) (27.9462, 4.3879) (27.9432, 4.3889) (27.9402, 4.39) (27.9373, 4.391) (27.9345, 4.392) (27.9318, 4.393) (27.9291, 4.3939) (27.9265, 4.3948) (27.9241, 4.3956) (27.9217, 4.3964) (27.9194, 4.3972) (27.9172, 4.398) (27.915, 4.3987) (27.913, 4.3993) (27.9111, 4.4) (27.9092, 4.4006) (27.9075, 4.4012) (27.9058, 4.4017) (27.9043, 4.4022) (27.9028, 4.4027) (27.9015, 4.4031) (27.9002, 4.4035) (27.8991, 4.4038) (27.898, 4.4042) (27.8971, 4.4044) (27.8963, 4.4047) (27.8956, 4.4049) (27.8951, 4.4051) (27.8948, 4.4052) (27.8946, 4.4052) (27.8945, 4.4052) knots -1 -1 -1 -1 -1 -1 -0.99583333 -0.99166667 -0.9875 -0.98333333 -0.97916667 -0.975 -0.97083333 -0.96666667 -0.9625 -0.95833333 -0.95416667 -0.95 -0.94583333 -0.94166667 -0.9375 -0.93333333 -0.92916667 -0.925 -0.92083333 -0.91666667 -0.9125 -0.90833333 -0.90416667 -0.9 -0.89583333 -0.89166667 -0.8875 -0.88333333 -0.87916667 -0.875 -0.87083333 -0.86666667 -0.8625 -0.85833333 -0.85416667 -0.85 -0.84583333 -0.84166667 -0.8375 -0.83333333 -0.82916667 -0.825 -0.82083333 -0.81666667 -0.8125 -0.80833333 -0.80416667 -0.8 -0.79583333 -0.79166667 -0.7875 -0.78333333 -0.77916667 -0.775 -0.77083333 -0.76666667 -0.7625 -0.75833333 -0.75416667 -0.75 -0.74583333 -0.74166667 -0.7375 -0.73333333 -0.72916667 -0.725 -0.72083333 -0.71666667 -0.7125 -0.70833333 -0.70416667 -0.7 -0.69583333 -0.69166667 -0.6875 -0.68333333 -0.67916667 -0.675 -0.67083333 -0.66666667 -0.6625 -0.65833333 -0.65416667 -0.65 -0.64583333 -0.64166667 -0.6375 -0.63333333 -0.62916667 -0.625 -0.62083333 -0.61666667 -0.6125 -0.60833333 -0.60416667 -0.6 -0.59583333 -0.59166667 -0.5875 -0.58333333 -0.57916667 -0.575 -0.57083333 -0.56666667 -0.5625 -0.55833333 -0.55416667 -0.55 -0.54583333 -0.54166667 -0.5375 -0.53333333 -0.52916667 -0.525 -0.52083333 -0.51666667 -0.5125 -0.50833333 -0.50416667 -0.5 -0.49583333 -0.49166667 -0.4875 -0.48333333 -0.47916667 -0.475 -0.47083333 -0.46666667 -0.4625 -0.45833333 -0.45416667 -0.45 -0.44583333 -0.44166667 -0.4375 -0.43333333 -0.42916667 -0.425 -0.42083333 -0.41666667 -0.4125 -0.40833333 -0.40416667 -0.4 -0.39583333 -0.39166667 -0.3875 -0.38333333 -0.37916667 -0.375 -0.37083333 -0.36666667 -0.3625 -0.35833333 -0.35416667 -0.35 -0.34583333 -0.34166667 -0.3375 -0.33333333 -0.32916667 -0.325 -0.32083333 -0.31666667 -0.3125 -0.30833333 -0.30416667 -0.3 -0.29583333 -0.29166667 -0.2875 -0.28333333 -0.27916667 -0.275 -0.27083333 -0.26666667 -0.2625 -0.25833333 -0.25416667 -0.25 -0.24583333 -0.24166667 -0.2375 -0.23333333 -0.22916667 -0.225 -0.22083333 -0.21666667 -0.2125 -0.20833333 -0.20416667 -0.2 -0.19583333 -0.19166667 -0.1875 -0.18333333 -0.17916667 -0.175 -0.17083333 -0.16666667 -0.1625 -0.15833333 -0.15416667 -0.15 -0.14583333 -0.14166667 -0.1375 -0.13333333 -0.12916667 -0.125 -0.12083333 -0.11666667 -0.1125 -0.10833333 -0.10416667 -0.1 -0.09583333 -0.09166667 -0.0875 -0.08333333 -0.07916667 -0.075 -0.07083333 -0.06666667 -0.0625 -0.05833333 -0.05416667 -0.05 -0.04583333 -0.04166667 -0.0375 -0.03333333 -0.02916667 -0.025 -0.02083333 -0.01666667 -0.0125 -0.00833333 -0.00416667 0 0 0 0 0 0
  line L39 (10.8547, -14.1221) -> (10.9659, -14.3948)
  arc A23 (27.6109, 4.4875) -> (27.918, 5.6335) centre (0, 12.5) ccw
  line L40 (9.8469, -14.8243) -> (9.7471, -14.5473)
  line L41 (10.9659, -14.3948) -> (10.9662, -14.3955)
  line L42 (5.1346, 41.0878) -> (5.1345, 41.087)
  line L43 (-0.9119, -16.2355) -> (-0.9213, -16.5298)
  spline S9 degree 5 poles (12.1618, 41.0147) (12.16, 41.0128) (12.1562, 41.0089) (12.1506, 41.003) (12.1432, 40.9951) (12.134, 40.9854) (12.1248, 40.9756) (12.1156, 40.9658) (12.1065, 40.9561) (12.0973, 40.9464) (12.0883, 40.9366) (12.0792, 40.9269) (12.0702, 40.9172) (12.0613, 40.9075) (12.0523, 40.8978) (12.0434, 40.8882) (12.0345, 40.8785) (12.0257, 40.8689) (12.0169, 40.8593) (12.0081, 40.8496) (11.9994, 40.84) (11.9907, 40.8305) (11.982, 40.8209) (11.9734, 40.8113) (11.9648, 40.8018) (11.9562, 40.7922) (11.9477, 40.7827) (11.9392, 40.7732) (11.9307, 40.7637) (11.9223, 40.7542) (11.9139, 40.7447) (11.9055, 40.7353) (11.8972, 40.7259) (11.8889, 40.7164) (11.8807, 40.707) (11.8724, 40.6976) (11.8643, 40.6882) (11.8561, 40.6789) (11.848, 40.6695) (11.8399, 40.6602) (11.8318, 40.6509) (11.8238, 40.6416) (11.8158, 40.6323) (11.8079, 40.623) (11.8, 40.6137) (11.7921, 40.6045) (11.7843, 40.5953) (11.7765, 40.5861) (11.7687, 40.5769) (11.7609, 40.5677) (11.7532, 40.5585) (11.7456, 40.5494) (11.7379, 40.5403) (11.7303, 40.5312) (11.7228, 40.5221) (11.7153, 40.513) (11.7078, 40.5039) (11.7003, 40.4949) (11.6929, 40.4859) (11.6855, 40.4769) (11.6781, 40.4679) (11.6708, 40.4589) (11.6635, 40.45) (11.6563, 40.4411) (11.6491, 40.4322) (11.6419, 40.4233) (11.6348, 40.4144) (11.6276, 40.4055) (11.6206, 40.3967) (11.6135, 40.3879) (11.6065, 40.3791) (11.5996, 40.3704) (11.5927, 40.3616) (11.5858, 40.3529) (11.5789, 40.3442) (11.5721, 40.3355) (11.5653, 40.3268) (11.5585, 40.3182) (11.5518, 40.3096) (11.5452, 40.301) (11.5385, 40.2924) (11.5319, 40.2838) (11.5253, 40.2753) (11.5188, 40.2668) (11.5123, 40.2583) (11.5058, 40.2498) (11.4994, 40.2414) (11.493, 40.233) (11.4867, 40.2246) (11.4803, 40.2162) (11.4741, 40.2078) (11.4678, 40.1995) (11.4616, 40.1912) (11.4554, 40.1829) (11.4493, 40.1747) (11.4432, 40.1665) (11.4371, 40.1582) (11.4311, 40.1501) (11.4251, 40.1419) (11.4192, 40.1338) (11.4132, 40.1257) (11.4074, 40.1176) (11.4015, 40.1096) (11.3957, 40.1015) (11.3899, 40.0936) (11.3842, 40.0856) (11.3785, 40.0776) (11.3728, 40.0697) (11.3672, 40.0618) (11.3616, 40.054) (11.3561, 40.0462) (11.3506, 40.0384) (11.3451, 40.0306) (11.3396, 40.0228) (11.3342, 40.0151) (11.3289, 40.0074) (11.3235, 39.9998) (11.3183, 39.9922) (11.313, 39.9846) (11.3078, 39.977) (11.3026, 39.9695) (11.2975, 39.962) (11.2924, 39.9545) (11.2873, 39.947) (11.2823, 39.9396) (11.2773, 39.9323) (11.2723, 39.9249) (11.2674, 39.9176) (11.2625, 39.9103) (11.2577, 39.9031) (11.2529, 39.8958) (11.2481, 39.8887) (11.2434, 39.8815) (11.2387, 39.8744) (11.234, 39.8673) (11.2294, 39.8603) (11.2248, 39.8533) (11.2203, 39.8463) (11.2158, 39.8393) (11.2113, 39.8324) (11.2069, 39.8256) (11.2025, 39.8187) (11.1982, 39.8119) (11.1939, 39.8052) (11.1896, 39.7985) (11.1854, 39.7918) (11.1812, 39.7851) (11.177, 39.7785) (11.1729, 39.772) (11.1688, 39.7654) (11.1648, 39.759) (11.1608, 39.7525) (11.1568, 39.7461) (11.1529, 39.7397) (11.149, 39.7334) (11.1451, 39.7271) (11.1413, 39.7209) (11.1376, 39.7147) (11.1338, 39.7085) (11.1301, 39.7024) (11.1265, 39.6963) (11.1229, 39.6903) (11.1193, 39.6843) (11.1158, 39.6784) (11.1123, 39.6725) (11.1088, 39.6666) (11.1054, 39.6608) (11.102, 39.655) (11.0987, 39.6493) (11.0954, 39.6436) (11.0921, 39.638) (11.0889, 39.6324) (11.0857, 39.6269) (11.0826, 39.6214) (11.0795, 39.616) (11.0764, 39.6106) (11.0734, 39.6053) (11.0704, 39.6) (11.0675, 39.5948) (11.0646, 39.5896) (11.0617, 39.5845) (11.0589, 39.5794) (11.0561, 39.5744) (11.0534, 39.5694) (11.0507, 39.5645) (11.048, 39.5597) (11.0454, 39.5549) (11.0428, 39.5501) (11.0403, 39.5454) (11.0378, 39.5408) (11.0353, 39.5362) (11.0329, 39.5317) (11.0306, 39.5272) (11.0282, 39.5228) (11.0259, 39.5185) (11.0237, 39.5142) (11.0215, 39.51) (11.0193, 39.5058) (11.0172, 39.5017) (11.0151, 39.4977) (11.0131, 39.4937) (11.0111, 39.4898) (11.0091, 39.486) (11.0072, 39.4822) (11.0053, 39.4785) (11.0035, 39.4748) (11.0017, 39.4713) (10.9999, 39.4678) (10.9982, 39.4643) (10.9966, 39.461) (10.9949, 39.4577) (10.9934, 39.4544) (10.9918, 39.4513) (10.9903, 39.4482) (10.9889, 39.4452) (10.9875, 39.4423) (10.9861, 39.4394) (10.9848, 39.4366) (10.9835, 39.4339) (10.9823, 39.4313) (10.9811, 39.4288) (10.9799, 39.4263) (10.9788, 39.424) (10.9778, 39.4217) (10.9768, 39.4195) (10.9758, 39.4173) (10.9749, 39.4153) (10.974, 39.4134) (10.9731, 39.4115) (10.9724, 39.4097) (10.9716, 39.408) (10.9709, 39.4065) (10.9702, 39.405) (10.9696, 39.4036) (10.9691, 39.4023) (10.9685, 39.4011) (10.9681, 39.4) (10.9676, 39.399) (10.9672, 39.3981) (10.9669, 39.3973) (10.9666, 39.3966) (10.9664, 39.3961) (10.9663, 39.3958) (10.9662, 39.3956) (10.9662, 39.3955) knots -1 -1 -1 -1 -1 -1 -0.99583333 -0.99166667 -0.9875 -0.98333333 -0.97916667 -0.975 -0.97083333 -0.96666667 -0.9625 -0.95833333 -0.95416667 -0.95 -0.94583333 -0.94166667 -0.9375 -0.93333333 -0.92916667 -0.925 -0.92083333 -0.91666667 -0.9125 -0.90833333 -0.90416667 -0.9 -0.89583333 -0.89166667 -0.8875 -0.88333333 -0.87916667 -0.875 -0.87083333 -0.86666667 -0.8625 -0.85833333 -0.85416667 -0.85 -0.84583333 -0.84166667 -0.8375 -0.83333333 -0.82916667 -0.825 -0.82083333 -0.81666667 -0.8125 -0.80833333 -0.80416667 -0.8 -0.79583333 -0.79166667 -0.7875 -0.78333333 -0.77916667 -0.775 -0.77083333 -0.76666667 -0.7625 -0.75833333 -0.75416667 -0.75 -0.74583333 -0.74166667 -0.7375 -0.73333333 -0.72916667 -0.725 -0.72083333 -0.71666667 -0.7125 -0.70833333 -0.70416667 -0.7 -0.69583333 -0.69166667 -0.6875 -0.68333333 -0.67916667 -0.675 -0.67083333 -0.66666667 -0.6625 -0.65833333 -0.65416667 -0.65 -0.64583333 -0.64166667 -0.6375 -0.63333333 -0.62916667 -0.625 -0.62083333 -0.61666667 -0.6125 -0.60833333 -0.60416667 -0.6 -0.59583333 -0.59166667 -0.5875 -0.58333333 -0.57916667 -0.575 -0.57083333 -0.56666667 -0.5625 -0.55833333 -0.55416667 -0.55 -0.54583333 -0.54166667 -0.5375 -0.53333333 -0.52916667 -0.525 -0.52083333 -0.51666667 -0.5125 -0.50833333 -0.50416667 -0.5 -0.49583333 -0.49166667 -0.4875 -0.48333333 -0.47916667 -0.475 -0.47083333 -0.46666667 -0.4625 -0.45833333 -0.45416667 -0.45 -0.44583333 -0.44166667 -0.4375 -0.43333333 -0.42916667 -0.425 -0.42083333 -0.41666667 -0.4125 -0.40833333 -0.40416667 -0.4 -0.39583333 -0.39166667 -0.3875 -0.38333333 -0.37916667 -0.375 -0.37083333 -0.36666667 -0.3625 -0.35833333 -0.35416667 -0.35 -0.34583333 -0.34166667 -0.3375 -0.33333333 -0.32916667 -0.325 -0.32083333 -0.31666667 -0.3125 -0.30833333 -0.30416667 -0.3 -0.29583333 -0.29166667 -0.2875 -0.28333333 -0.27916667 -0.275 -0.27083333 -0.26666667 -0.2625 -0.25833333 -0.25416667 -0.25 -0.24583333 -0.24166667 -0.2375 -0.23333333 -0.22916667 -0.225 -0.22083333 -0.21666667 -0.2125 -0.20833333 -0.20416667 -0.2 -0.19583333 -0.19166667 -0.1875 -0.18333333 -0.17916667 -0.175 -0.17083333 -0.16666667 -0.1625 -0.15833333 -0.15416667 -0.15 -0.14583333 -0.14166667 -0.1375 -0.13333333 -0.12916667 -0.125 -0.12083333 -0.11666667 -0.1125 -0.10833333 -0.10416667 -0.1 -0.09583333 -0.09166667 -0.0875 -0.08333333 -0.07916667 -0.075 -0.07083333 -0.06666667 -0.0625 -0.05833333 -0.05416667 -0.05 -0.04583333 -0.04166667 -0.0375 -0.03333333 -0.02916667 -0.025 -0.02083333 -0.01666667 -0.0125 -0.00833333 -0.00416667 0 0 0 0 0 0
  line L44 (28.587, 7.3655) -> (28.2972, 7.4176)